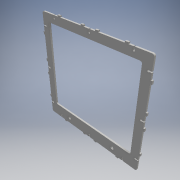
# Autodesk Inventor part: painel superior
Saved by Autodesk Inventor 2016 (Build 200138000, 138)
## iProperties
Created: 2016-08-08
Part Number: painel superior
Material: Generic
Document SubType Name: Modeling
Designer: Waldo
Density: 1 g/cm^3
Appearance: Default
Author: Waldo
Autodesk Inventor part; units mm, degrees
ref_plane "YZ Plane" through (0, 0, 0) normal (1, 0, 0) x (0, 1, 0)
ref_plane "XZ Plane" through (0, 0, 0) normal (0, 1, 0) x (-1, 0, 0)
ref_plane "XY Plane" through (0, 0, 0) normal (0, 0, 1) x (1, 0, 0)
sketch "Sketch1" plane through (0, 0, 0) normal (0, 1, 0) x (-1, 0, 0)
  circle A0 centre (93, -346) radius 6
  circle A1 centre (283, -346) radius 6
  line L0 (349, -33) -> (349, -313.9794)
  arc A2 (342.9794, -320) -> (349, -313.9794) centre (342.9794, -313.9794) ccw
  line L1 (342.9794, -320) -> (33.0419, -320)
  arc A3 (27, -313.9581) -> (33.0419, -320) centre (33.0419, -313.9581) ccw
  line L2 (27, -313.9581) -> (27, -33)
  arc A4 (33, -27) -> (27, -33) centre (33, -33) ccw
  line L3 (33, -27) -> (343, -27)
  arc A5 (349, -33) -> (343, -27) centre (343, -33) ccw
  arc A6 (53.2, -360.4998) -> (54.4903, -358.9717) centre (52.9403, -358.9717) ccw
  line L4 (53.2, -367) -> (53.2, -360.4998)
  line L5 (67.5, -367) -> (53.2, -367)
  line L6 (67.5, -371.5) -> (67.5, -367)
  line L7 (77.5, -371.5) -> (67.5, -371.5)
  line L8 (77.5, -367) -> (77.5, -371.5)
  line L9 (158, -367) -> (77.5, -367)
  line L10 (158, -371.5) -> (158, -367)
  line L11 (168, -371.5) -> (158, -371.5)
  line L12 (168, -367) -> (168, -371.5)
  line L13 (186.45, -367) -> (168, -367)
  line L14 (186.45, -360.4998) -> (186.45, -367)
  arc A7 (185.1597, -358.9717) -> (186.45, -360.4998) centre (186.7097, -358.9717) ccw
  line L15 (185.1597, -357.4217) -> (185.1597, -358.9717)
  arc A8 (185.8652, -356.1219) -> (185.1597, -357.4217) centre (186.7097, -357.4217) ccw
  line L16 (186.0345, -356.1219) -> (185.8652, -356.1219)
  arc A9 (189.9655, -356.1219) -> (186.0345, -356.1219) centre (188, -356.8524) ccw
  line L17 (190.1348, -356.1219) -> (189.9655, -356.1219)
  arc A10 (190.8403, -357.4217) -> (190.1348, -356.1219) centre (189.2903, -357.4217) ccw
  line L18 (190.8403, -358.9717) -> (190.8403, -357.4217)
  arc A11 (189.55, -360.4998) -> (190.8403, -358.9717) centre (189.2903, -358.9717) ccw
  line L19 (189.55, -367) -> (189.55, -360.4998)
  line L20 (208, -367) -> (189.55, -367)
  line L21 (208, -371.5) -> (208, -367)
  line L22 (218, -371.5) -> (208, -371.5)
  line L23 (218, -367) -> (218, -371.5)
  line L24 (298.5, -367) -> (218, -367)
  line L25 (298.5, -371.5) -> (298.5, -367)
  line L26 (308.5, -371.5) -> (298.5, -371.5)
  line L27 (308.5, -367) -> (308.5, -371.5)
  line L28 (322.8019, -367) -> (308.5, -367)
  line L29 (322.8019, -360.4998) -> (322.8019, -367)
  arc A12 (321.5115, -358.9717) -> (322.8019, -360.4998) centre (323.0615, -358.9717) ccw
  line L30 (321.5115, -357.4217) -> (321.5115, -358.9717)
  arc A13 (322.2171, -356.1219) -> (321.5115, -357.4217) centre (323.0615, -357.4217) ccw
  line L31 (322.3864, -356.1219) -> (322.2171, -356.1219)
  arc A14 (326.3174, -356.1219) -> (322.3864, -356.1219) centre (324.3519, -356.8524) ccw
  line L32 (326.4866, -356.1219) -> (326.3174, -356.1219)
  arc A15 (327.1922, -357.4217) -> (326.4866, -356.1219) centre (325.6422, -357.4217) ccw
  line L33 (327.1922, -358.9717) -> (327.1922, -357.4217)
  arc A16 (325.9019, -360.4998) -> (327.1922, -358.9717) centre (325.6422, -358.9717) ccw
  line L34 (325.9019, -367) -> (325.9019, -360.4998)
  line L35 (370, -367) -> (325.9019, -367)
  arc A17 (370, -367) -> (376, -361) centre (370, -361) ccw
  line L36 (376, -325.25) -> (376, -361)
  line L37 (369.4998, -325.25) -> (376, -325.25)
  arc A18 (367.9717, -326.5403) -> (369.4998, -325.25) centre (367.9717, -324.9903) ccw
  line L38 (366.4217, -326.5403) -> (367.9717, -326.5403)
  arc A19 (365.1219, -325.8348) -> (366.4217, -326.5403) centre (366.4217, -324.9903) ccw
  line L39 (365.1219, -325.6655) -> (365.1219, -325.8348)
  arc A20 (365.1219, -321.7345) -> (365.1219, -325.6655) centre (365.8524, -323.7) ccw
  line L40 (365.1219, -321.5652) -> (365.1219, -321.7345)
  arc A21 (366.4217, -320.8597) -> (365.1219, -321.5652) centre (366.4217, -322.4097) ccw
  line L41 (367.9717, -320.8597) -> (366.4217, -320.8597)
  arc A22 (369.4998, -322.15) -> (367.9717, -320.8597) centre (367.9717, -322.4097) ccw
  line L42 (376, -322.15) -> (369.4998, -322.15)
  line L43 (376, -304.2) -> (376, -322.15)
  line L44 (380.5, -304.2) -> (376, -304.2)
  line L45 (380.5, -294.2) -> (380.5, -304.2)
  line L46 (376, -294.2) -> (380.5, -294.2)
  line L47 (376, -213.5) -> (376, -294.2)
  line L48 (380.5, -213.5) -> (376, -213.5)
  line L49 (380.5, -203.5) -> (380.5, -213.5)
  line L50 (376, -203.5) -> (380.5, -203.5)
  line L51 (376, -184.7642) -> (376, -203.5)
  line L52 (369.4998, -184.7642) -> (376, -184.7642)
  arc A23 (367.9717, -186.0545) -> (369.4998, -184.7642) centre (367.9717, -184.5045) ccw
  line L53 (366.4217, -186.0545) -> (367.9717, -186.0545)
  arc A24 (365.1219, -185.349) -> (366.4217, -186.0545) centre (366.4217, -184.5045) ccw
  line L54 (365.1219, -185.1797) -> (365.1219, -185.349)
  arc A25 (365.1219, -181.2487) -> (365.1219, -185.1797) centre (365.8524, -183.2142) ccw
  line L55 (365.1219, -181.0794) -> (365.1219, -181.2487)
  arc A26 (366.4217, -180.3739) -> (365.1219, -181.0794) centre (366.4217, -181.9239) ccw
  line L56 (367.9717, -180.3739) -> (366.4217, -180.3739)
  arc A27 (369.4998, -181.6642) -> (367.9717, -180.3739) centre (367.9717, -181.9239) ccw
  line L57 (376, -181.6642) -> (369.4998, -181.6642)
  line L58 (376, -163.5) -> (376, -181.6642)
  line L59 (380.5, -163.5) -> (376, -163.5)
  line L60 (380.5, -153.5) -> (380.5, -163.5)
  line L61 (376, -153.5) -> (380.5, -153.5)
  line L62 (376, -72.8) -> (376, -153.5)
  line L63 (380.5, -72.8) -> (376, -72.8)
  line L64 (380.5, -62.8) -> (380.5, -72.8)
  line L65 (376, -62.8) -> (380.5, -62.8)
  line L66 (376, -44.278) -> (376, -62.8)
  line L67 (369.4998, -44.278) -> (376, -44.278)
  arc A28 (367.9717, -45.5683) -> (369.4998, -44.278) centre (367.9717, -44.0183) ccw
  line L68 (366.4217, -45.5683) -> (367.9717, -45.5683)
  arc A29 (365.1219, -44.8627) -> (366.4217, -45.5683) centre (366.4217, -44.0183) ccw
  line L69 (365.1219, -44.6935) -> (365.1219, -44.8627)
  arc A30 (365.1219, -40.7625) -> (365.1219, -44.6935) centre (365.8524, -42.728) ccw
  line L70 (365.1219, -40.5932) -> (365.1219, -40.7625)
  arc A31 (366.4217, -39.8876) -> (365.1219, -40.5932) centre (366.4217, -41.4376) ccw
  line L71 (367.9717, -39.8876) -> (366.4217, -39.8876)
  arc A32 (369.4998, -41.178) -> (367.9717, -39.8876) centre (367.9717, -41.4376) ccw
  line L72 (376, -41.178) -> (369.4998, -41.178)
  line L73 (376, -6) -> (376, -41.178)
  arc A33 (376, -6) -> (370, 0) centre (370, -6) ccw
  line L74 (325.9019, 0) -> (370, 0)
  line L75 (325.9019, -6.5002) -> (325.9019, 0)
  arc A34 (327.1922, -8.0283) -> (325.9019, -6.5002) centre (325.6422, -8.0283) ccw
  line L76 (327.1922, -9.5783) -> (327.1922, -8.0283)
  arc A35 (326.4866, -10.8781) -> (327.1922, -9.5783) centre (325.6422, -9.5783) ccw
  line L77 (326.3174, -10.8781) -> (326.4866, -10.8781)
  arc A36 (322.3864, -10.8781) -> (326.3174, -10.8781) centre (324.3519, -10.1476) ccw
  line L78 (322.2171, -10.8781) -> (322.3864, -10.8781)
  arc A37 (321.5115, -9.5783) -> (322.2171, -10.8781) centre (323.0615, -9.5783) ccw
  line L79 (321.5115, -8.0283) -> (321.5115, -9.5783)
  arc A38 (322.8019, -6.5002) -> (321.5115, -8.0283) centre (323.0615, -8.0283) ccw
  line L80 (322.8019, 0) -> (322.8019, -6.5002)
  line L81 (308.5, 0) -> (322.8019, 0)
  line L82 (308.5, 4.5) -> (308.5, 0)
  line L83 (298.5, 4.5) -> (308.5, 4.5)
  line L84 (298.5, 0) -> (298.5, 4.5)
  line L85 (218, 0) -> (298.5, 0)
  line L86 (218, 4.5) -> (218, 0)
  line L87 (208, 4.5) -> (218, 4.5)
  line L88 (208, 0) -> (208, 4.5)
  line L89 (189.55, 0) -> (208, 0)
  line L90 (189.55, -6.5002) -> (189.55, 0)
  arc A39 (190.8403, -8.0283) -> (189.55, -6.5002) centre (189.2903, -8.0283) ccw
  line L91 (190.8403, -9.5783) -> (190.8403, -8.0283)
  arc A40 (190.1348, -10.8781) -> (190.8403, -9.5783) centre (189.2903, -9.5783) ccw
  line L92 (189.9655, -10.8781) -> (190.1348, -10.8781)
  arc A41 (186.0345, -10.8781) -> (189.9655, -10.8781) centre (188, -10.1476) ccw
  line L93 (185.8652, -10.8781) -> (186.0345, -10.8781)
  arc A42 (185.1597, -9.5783) -> (185.8652, -10.8781) centre (186.7097, -9.5783) ccw
  line L94 (185.1597, -8.0283) -> (185.1597, -9.5783)
  arc A43 (186.45, -6.5002) -> (185.1597, -8.0283) centre (186.7097, -8.0283) ccw
  line L95 (186.45, 0) -> (186.45, -6.5002)
  line L96 (168, 0) -> (186.45, 0)
  line L97 (168, 4.5) -> (168, 0)
  line L98 (158, 4.5) -> (168, 4.5)
  line L99 (158, 0) -> (158, 4.5)
  line L100 (77.5, 0) -> (158, 0)
  line L101 (77.5, 4.5) -> (77.5, 0)
  line L102 (67.5, 4.5) -> (77.5, 4.5)
  line L103 (67.5, 0) -> (67.5, 4.5)
  line L104 (53.2, 0) -> (67.5, 0)
  line L105 (53.2, -6.5002) -> (53.2, 0)
  arc A44 (54.4903, -8.0283) -> (53.2, -6.5002) centre (52.9403, -8.0283) ccw
  line L106 (54.4903, -9.5783) -> (54.4903, -8.0283)
  arc A45 (53.7848, -10.8781) -> (54.4903, -9.5783) centre (52.9403, -9.5783) ccw
  line L107 (53.6155, -10.8781) -> (53.7848, -10.8781)
  arc A46 (49.6845, -10.8781) -> (53.6155, -10.8781) centre (51.65, -10.1476) ccw
  line L108 (49.5152, -10.8781) -> (49.6845, -10.8781)
  arc A47 (48.8097, -9.5783) -> (49.5152, -10.8781) centre (50.3597, -9.5783) ccw
  line L109 (48.8097, -8.0283) -> (48.8097, -9.5783)
  arc A48 (50.1, -6.5002) -> (48.8097, -8.0283) centre (50.3597, -8.0283) ccw
  line L110 (50.1, 0) -> (50.1, -6.5002)
  line L111 (6, 0) -> (50.1, 0)
  arc A49 (6, 0) -> (0, -6) centre (6, -6) ccw
  line L112 (0, -41.3) -> (0, -6)
  line L113 (6.5002, -41.3) -> (0, -41.3)
  arc A50 (8.0283, -40.0097) -> (6.5002, -41.3) centre (8.0283, -41.5597) ccw
  line L114 (9.5783, -40.0097) -> (8.0283, -40.0097)
  arc A51 (10.8781, -40.7152) -> (9.5783, -40.0097) centre (9.5783, -41.5597) ccw
  line L115 (10.8781, -40.8845) -> (10.8781, -40.7152)
  arc A52 (10.8781, -44.8155) -> (10.8781, -40.8845) centre (10.1476, -42.85) ccw
  line L116 (10.8781, -44.9848) -> (10.8781, -44.8155)
  arc A53 (9.5783, -45.6903) -> (10.8781, -44.9848) centre (9.5783, -44.1403) ccw
  line L117 (8.0283, -45.6903) -> (9.5783, -45.6903)
  arc A54 (6.5002, -44.4) -> (8.0283, -45.6903) centre (8.0283, -44.1403) ccw
  line L118 (0, -44.4) -> (6.5002, -44.4)
  line L119 (0, -62.8) -> (0, -44.4)
  line L120 (-4.5, -62.8) -> (0, -62.8)
  line L121 (-4.5, -72.8) -> (-4.5, -62.8)
  line L122 (0, -72.8) -> (-4.5, -72.8)
  line L123 (0, -153.5) -> (0, -72.8)
  line L124 (-4.5, -153.5) -> (0, -153.5)
  line L125 (-4.5, -163.5) -> (-4.5, -153.5)
  line L126 (0, -163.5) -> (-4.5, -163.5)
  line L127 (0, -181.85) -> (0, -163.5)
  line L128 (6.5002, -181.85) -> (0, -181.85)
  arc A55 (8.0283, -180.5597) -> (6.5002, -181.85) centre (8.0283, -182.1097) ccw
  line L129 (9.5783, -180.5597) -> (8.0283, -180.5597)
  arc A56 (10.8781, -181.2652) -> (9.5783, -180.5597) centre (9.5783, -182.1097) ccw
  line L130 (10.8781, -181.4345) -> (10.8781, -181.2652)
  arc A57 (10.8781, -185.3655) -> (10.8781, -181.4345) centre (10.1476, -183.4) ccw
  line L131 (10.8781, -185.5348) -> (10.8781, -185.3655)
  arc A58 (9.5783, -186.2403) -> (10.8781, -185.5348) centre (9.5783, -184.6903) ccw
  line L132 (8.0283, -186.2403) -> (9.5783, -186.2403)
  arc A59 (6.5002, -184.95) -> (8.0283, -186.2403) centre (8.0283, -184.6903) ccw
  line L133 (0, -184.95) -> (6.5002, -184.95)
  line L134 (0, -203.5) -> (0, -184.95)
  line L135 (-4.5, -203.5) -> (0, -203.5)
  line L136 (-4.5, -213.5) -> (-4.5, -203.5)
  line L137 (0, -213.5) -> (-4.5, -213.5)
  line L138 (0, -294.2) -> (0, -213.5)
  line L139 (-4.5, -294.2) -> (0, -294.2)
  line L140 (-4.5, -304.2) -> (-4.5, -294.2)
  line L141 (0, -304.2) -> (-4.5, -304.2)
  line L142 (0, -322.3349) -> (0, -304.2)
  line L143 (6.5002, -322.3349) -> (0, -322.3349)
  arc A60 (8.0283, -321.0445) -> (6.5002, -322.3349) centre (8.0283, -322.5945) ccw
  line L144 (9.5783, -321.0445) -> (8.0283, -321.0445)
  arc A61 (10.8781, -321.7501) -> (9.5783, -321.0445) centre (9.5783, -322.5945) ccw
  line L145 (10.8781, -321.9194) -> (10.8781, -321.7501)
  arc A62 (10.8781, -325.8504) -> (10.8781, -321.9194) centre (10.1476, -323.8849) ccw
  line L146 (10.8781, -326.0196) -> (10.8781, -325.8504)
  arc A63 (9.5783, -326.7252) -> (10.8781, -326.0196) centre (9.5783, -325.1752) ccw
  line L147 (8.0283, -326.7252) -> (9.5783, -326.7252)
  arc A64 (6.5002, -325.4349) -> (8.0283, -326.7252) centre (8.0283, -325.1752) ccw
  line L148 (0, -325.4349) -> (6.5002, -325.4349)
  line L149 (0, -361) -> (0, -325.4349)
  arc A65 (0, -361) -> (6, -367) centre (6, -361) ccw
  line L150 (50.1, -367) -> (6, -367)
  line L151 (50.1, -360.4998) -> (50.1, -367)
  arc A66 (48.8097, -358.9717) -> (50.1, -360.4998) centre (50.3597, -358.9717) ccw
  line L152 (48.8097, -357.4217) -> (48.8097, -358.9717)
  arc A67 (49.5152, -356.1219) -> (48.8097, -357.4217) centre (50.3597, -357.4217) ccw
  line L153 (49.6845, -356.1219) -> (49.5152, -356.1219)
  arc A68 (53.6155, -356.1219) -> (49.6845, -356.1219) centre (51.65, -356.8524) ccw
  line L154 (53.7848, -356.1219) -> (53.6155, -356.1219)
  arc A69 (54.4903, -357.4217) -> (53.7848, -356.1219) centre (52.9403, -357.4217) ccw
  line L155 (54.4903, -358.9717) -> (54.4903, -357.4217)
  point P0 (0, 0)
  constraints: 312 end point, 136 point on circle, 125 tangent, 86 parallel, 70 centre point, 65 equal radius, 40 perpendicular, 2 collinear
extrude "Extrusion1" add sketch "Sketch1" along normal blind 6
body "Solid1"
